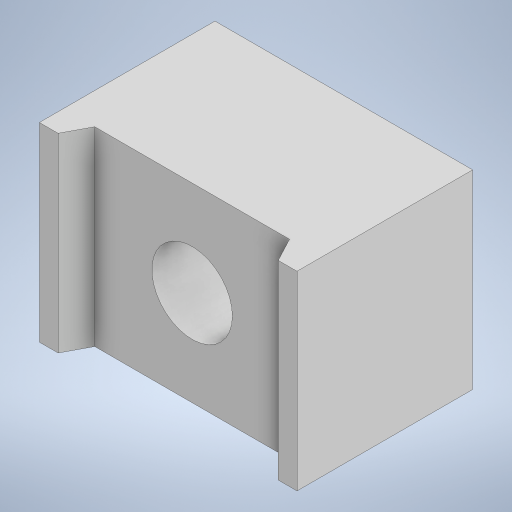
# Autodesk Inventor part: base_thorlabs
Saved by Autodesk Inventor 2024.2 (Build 282272000, 272)
## iProperties
Created: 2021-12-13
Part Number: base_thorlabs
Material: Generic
Document SubType Name: Modeling
Designer: magoo
Density: 1 g/cm^3
Appearance: Default
Description: 3D printing model
Author: magoo
Autodesk Inventor part; units mm, degrees
ref_plane "YZ Plane" through (0, 0, 0) normal (1, 0, 0) x (0, 1, 0)
ref_plane "XZ Plane" through (0, 0, 0) normal (0, 1, 0) x (-1, 0, 0)
ref_plane "XY Plane" through (0, 0, 0) normal (0, 0, 1) x (1, 0, 0)
sketch "Sketch1" plane through (0, 0, 0) normal (0, 0, 1) x (1, 0, 0)
  line L0 (6.88, -5.08) -> (-6.88, -5.08)
  line L1 (-6.88, -5.08) -> (-6.88, 5.08)
  line L2 (-6.88, 5.08) -> (6.88, 5.08)
  line L3 (6.88, 5.08) -> (6.88, -5.08)
  line L4 (6.88, -5.08) -> (-6.88, 5.08) construction
  line L5 (-6.88, -5.08) -> (6.88, 5.08) construction
  circle A0 centre (0, 0) radius 3.6
  circle A1 centre (0, 0) radius 2.15
  line L6 (6.88, 0) -> (-6.88, 0)
  line L7 (0, 5.08) -> (0, -5.08)
  dimension "d0" = 13.76
  dimension "d1" = 10.16
  dimension "d2" = 7.2
  dimension "d3" = 4.3
  constraints: 16 end point, 6 midpoint, 2 centre point, 2 coincident, 2 parallel, 1 horizontal, 1 perpendicular
  measures "d0" distance of L1.end L2.end
  measures "d1" distance of L0.end L1.end
  measures "d2" diameter of A0
  measures "d3" diameter of A1
extrude "Extrusion1" add sketch "Sketch1" along normal blind 9.379 contours L0 L7 A0 L6 L3 | L0 L1 L6 A0 L7 | L6 A0 L7 L2 L3 | L7 A1 L6 A0 | A0 L6 A1 L7 | L6 A1 L7 A0 | L1 L2 L7 A0 L6 | A0 L7 A1 L6
sketch "Sketch2" plane through (-6.88, 5.08, 0) normal (0, 1, 0) x (-1, 0, 0)
  line L0 (-12.08, 8.1) -> (-1.68, 8.1)
  line L1 (-6.88, 8.1) -> (-6.88, 9.379) construction
  line L2 (-13.76, 9.379) -> (0, 9.379) construction
  line L3 (-13.76, 9.379) -> (-12.76, 9.379)
  line L4 (0, 9.379) -> (-1, 9.379)
  line L5 (-12.08, 8.1) -> (-12.76, 9.379)
  line L6 (-1.68, 8.1) -> (-1, 9.379)
  line L7 (-13.76, 9.379) -> (-13.76, 11.379)
  line L8 (-13.76, 11.379) -> (0, 11.379)
  line L9 (0, 0) -> (0, 9.379) construction
  line L10 (0, 11.379) -> (0, 9.379)
  dimension "d6" = 10.4
  dimension "d19" = 1.279
  dimension "d20" = 1
  dimension "d21" = 1
  dimension "d22" = 2
  constraints: 18 end point, 3 horizontal, 2 midpoint, 2 vertical, 1 collinear, 1 perpendicular
  measures "d6" distance of L0.start L0.end
  measures "d19" distance of L1.start L1.end
  measures "d20" distance of L2.start L3.end
  measures "d21" distance of L2.end L4.end
  measures "d22" distance of L2.start L7.end
extrude "Extrusion2" cut sketch "Sketch2" against normal up to next
body "Solid1"
